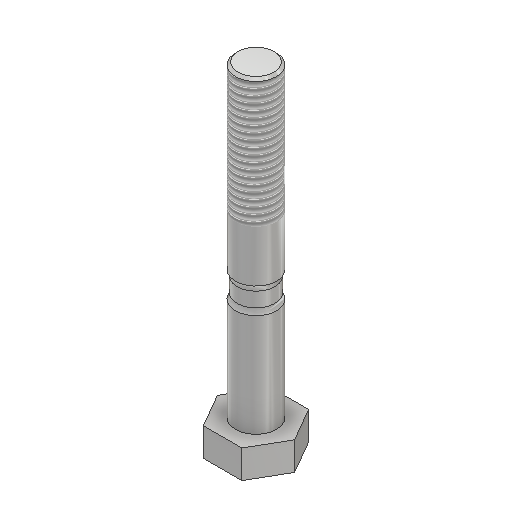
# Autodesk Inventor part: COTS_GENERIC_M8_Hobbed_Bolt
Saved by Autodesk Inventor 2026.1 (Build 301233000, 233)
## iProperties
Created: 2016-01-21
Part Number: COTS_GENERIC_M8_Hobbed_Bolt
Material: Ogólny
Document SubType Name: Modeling
Designer: Andrzej
Density: 1 g/cm^3
Appearance: Aluminium - ciemne
Mass: 3.78412 g
Surface Area: 20.3498 cm^2
Volume: 3.78412 cm^3
Author: Andrzej
Autodesk Inventor part; units mm, degrees
ref_plane "YZ Plane" through (0, 0, 0) normal (1, 0, 0) x (0, 1, 0)
ref_plane "XZ Plane" through (0, 0, 0) normal (0, 1, 0) x (-1, 0, 0)
ref_plane "XY Plane" through (0, 0, 0) normal (0, 0, 1) x (1, 0, 0)
sketch "Szkic1" plane through (0, 0, 0) normal (0, 0, 1) x (1, 0, 0)
  line L0 (3.7528, 6.5) -> (7.5056, 0)
  line L1 (7.5056, 0) -> (3.7528, -6.5)
  line L2 (3.7528, -6.5) -> (-3.7528, -6.5)
  line L3 (-3.7528, -6.5) -> (-7.5056, 0)
  line L4 (-7.5056, 0) -> (-3.7528, 6.5)
  line L5 (-3.7528, 6.5) -> (3.7528, 6.5)
  point P0 (0, 0)
  point P1 (0, 0)
  point P2 (0, 6.5)
  constraints: 12 end point, 1 midpoint, 13 other
extrude "Wyciągnięcie proste1" add sketch "Szkic1" along normal blind 5.5
sketch "Szkic2" plane through (0, 0, 5.5) normal (0, 0, 1) x (1, 0, 0)
  circle A0 centre (0, 0) radius 4
  dimension "d3" = 8
  constraints: 1 centre point, 1 coincident
  measures "d3" diameter of A0
extrude "Wyciągnięcie proste2" add sketch "Szkic2" along normal blind 20
sketch "Szkic3" plane through (0, 0, 25.5) normal (0, 0, 1) x (1, 0, 0)
  circle A0 centre (0, 0) radius 4 projected
  circle A1 centre (0, 0) radius 3.675
  dimension "d6" = 7.35
  constraints: 1 centre point, 1 coincident
  measures "d6" diameter of A1
extrude "Wyciągnięcie proste3" add sketch "Szkic3" along normal blind 5 contours A1
sketch "Szkic4" plane through (0, 0, 30.5) normal (0, 0, 1) x (1, 0, 0)
  circle A0 centre (0, 0) radius 4 projected
extrude "Wyciągnięcie proste4" add sketch "Szkic4" along normal blind 35
thread "Gwint1" size "M8x1.25" class "6g" standard "ANSI Metric M Profile" length 25 offset 10
fillet "Zaokrąglenie1" radius 2 2 edges at (-3.675, 0, 25.5) (-3.675, 0, 30.5)
chamfer "Faza1" distance 0.5 angle 45 1 edges at (-4, 0, 65.5)
